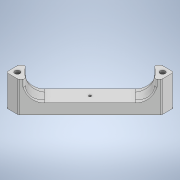
# Autodesk Inventor part: rotor_core
Saved by Autodesk Inventor 2021 (Build 250183000, 183)
## iProperties
Created: 2022-02-28
Part Number: rotor_core
Material: Generic
Document SubType Name: Modeling
Designer: ermoz
Density: 1 g/cm^3
Appearance: Default
Author: ermoz
Autodesk Inventor part; units mm, degrees
ref_plane "YZ Plane" through (0, 0, 0) normal (1, 0, 0) x (0, 1, 0)
ref_plane "XZ Plane" through (0, 0, 0) normal (0, 1, 0) x (-1, 0, 0)
ref_plane "XY Plane" through (0, 0, 0) normal (0, 0, 1) x (1, 0, 0)
sketch "Sketch1" plane through (0, 0, 0) normal (0, 1, 0) x (-1, 0, 0)
  line L0 (-12.5, -12.5) -> (12.5, -12.5)
  line L1 (12.5, -12.5) -> (12.5, 12.5)
  line L2 (12.5, 12.5) -> (-12.5, 12.5)
  line L3 (-12.5, 12.5) -> (-12.5, -12.5)
  line L4 (-12.5, -12.5) -> (12.5, 12.5) construction
  line L5 (12.5, -12.5) -> (-12.5, 12.5) construction
  line L6 (12.25, 12.25) -> (12.25, -12.25)
  line L7 (12.25, -12.25) -> (-12.25, -12.25)
  line L8 (-12.25, -12.25) -> (-12.25, 12.25)
  line L9 (-12.25, 12.25) -> (12.25, 12.25)
  circle A0 centre (0, 0) radius 13.5
  line L10 (-10.4822, -14.0178) -> (14.0178, 10.4822)
  line L11 (14.0178, 10.4822) -> (10.4822, 14.0178)
  line L12 (10.4822, 14.0178) -> (-14.0178, -10.4822)
  line L13 (-14.0178, -10.4822) -> (-10.4822, -14.0178)
  line L14 (-10.4822, -14.0178) -> (10.4822, 14.0178) construction
  line L15 (14.0178, 10.4822) -> (-14.0178, -10.4822) construction
  point P0 (-11.1486, -7.6131)
  point P1 (-12.25, -8.7145)
  point P2 (-8.7145, -12.25)
  point P3 (-7.6131, -11.1486)
  point P4 (8.7145, 12.25)
  point P5 (7.6131, 11.1486)
  point P6 (11.1486, 7.6131)
  point P7 (12.25, 8.7145)
  dimension "d0" = 25
  dimension "d1" = 25
  dimension "d2" = 0.25
  dimension "d3" = 27
  dimension "d4" = 5
  constraints: 32 end point, 7 parallel, 4 midpoint, 3 perpendicular, 1 centre point, 1 coincident, 1 horizontal, 3 other
  measures "d0" distance of L2.end L1.end
  measures "d1" distance of L1.end L0.end
  measures "d2" distance between parallel lines of L1 L6
  measures "d3" diameter of A0
  measures "d4" distance of L11.end L10.end
extrude "Extrusion1" add sketch "Sketch1" along normal blind 9 contours L8 L12 A0 L10 L7 | A0 L12 L9 L6 L10
extrude "Extrusion2" add sketch "Sketch1" along normal blind 3 contours A0 L12 L10
sketch "Sketch2" plane through (0, 3, 0) normal (0, 1, 0) x (1, 0, 0)
  circle A0 centre (0, 0) radius 0.35
  dimension "d9" = 0.7
  constraints: 1 centre point, 1 coincident
  measures "d9" diameter of A0
extrude "Extrusion3" cut sketch "Sketch2" against normal up to surface (3 mm away)
fillet "Fillet1" radius 0.5 10 edges at (12.25, 4.5, -12.25) (12.25, 4.5, -8.7145) (11.1486, 6, -7.6131) (7.6131, 6, -11.1486) (8.7145, 4.5, -12.25) (-7.6131, 6, 11.1486) (-11.1486, 6, 7.6131) (-12.25, 4.5, 8.7145) (-12.25, 4.5, 12.25) (-8.7145, 4.5, 12.25)
fillet "Fillet2" radius 4 6 edges at (-11.1764, 3, 7.885) (-7.885, 3, 11.1764) (-9.5459, 3, 9.5459) (11.1764, 3, -7.885) (7.885, 3, -11.1764) (9.5459, 3, -9.5459)
ref_plane "Work Plane2" through (9.5459, 0, -9.5459) normal (0.7071068, 0, -0.7071068) x (0, 1, 0)
ref_plane "Work Plane1" through (1.7678, 3, 1.7678) normal (0.7071068, 0, -0.7071068) x (0, 1, 0)
sketch "Sketch4" plane through (0, 9, 0) normal (0, 1, 0) x (1, 0, 0)
  line L0 (0, 0) -> (10.6066, 10.6066)
  line L1 (0, 0) -> (15, 0) construction
  circle A0 centre (0, 0) radius 0.35 projected
  line L2 (0, 0) -> (-10.6066, -10.6066)
  line L3 (0, 0) -> (15, 0) construction
  circle A1 centre (10.6066, 10.6066) radius 0.75
  circle A2 centre (-10.6066, -10.6066) radius 0.75
  dimension "d21" = 15
  dimension "d22" = 45
  dimension "d23" = 15
  dimension "d24" = 135
  dimension "d25" = 1.5
  constraints: 8 end point, 2 centre point, 2 coincident, 2 equal length, 2 horizontal, 1 equal radius
  measures "d21" distance of L0.start L0.end
  measures "d22" angle of L1 L0
  measures "d23" distance of L2.start L2.end
  measures "d24" angle of L2 L3
  measures "d25" diameter of A1
extrude "Extrusion5" cut sketch "Sketch4" against normal through all contours A1 | A2
body "Solid1"
